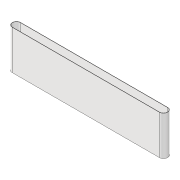
# Autodesk Inventor part: Band
Saved by Autodesk Inventor 2020 (Build 240168000, 168)
## iProperties
Created: 2020-03-18
Part Number: Band
Material: Generisch
Document SubType Name: Modeling
Designer: franz
Density: 1 g/cm^3
Appearance: Vorgabe
Author: franz
Autodesk Inventor part; units mm, degrees
ref_plane "YZ Plane" through (0, 0, 0) normal (1, 0, 0) x (0, 1, 0)
ref_plane "XZ Plane" through (0, 0, 0) normal (0, 1, 0) x (-1, 0, 0)
ref_plane "XY Plane" through (0, 0, 0) normal (0, 0, 1) x (1, 0, 0)
sketch "Skizze1" plane through (0, 0, 0) normal (0, 1, 0) x (-1, 0, 0)
  arc A0 (0, -40) -> (0, 40) centre (0, 0) ccw
  arc A1 (0, -43) -> (0, 43) centre (0, 0) ccw
  arc A2 (-1500, 40) -> (-1500, -40) centre (-1500, 0) ccw
  arc A3 (-1500, 43) -> (-1500, -43) centre (-1500, 0) ccw
  line L0 (0, 43) -> (-1500, 43)
  line L1 (-1500, 40) -> (0, 40)
  line L2 (0, -40) -> (-1500, -40)
  line L3 (-1500, -43) -> (0, -43)
  dimension "d0" = 80
  dimension "d1" = 86
  dimension "d2" = 80
  dimension "d3" = 86
  dimension "d4" = 1500
  constraints: 12 point on circle, 8 end point, 4 centre point, 4 coincident, 4 point on line, 4 tangent, 3 parallel, 1 horizontal
  measures "d0" diameter of A0
  measures "d1" diameter of A1
  measures "d2" diameter of A2
  measures "d3" diameter of A3
  measures "d4" distance of point (-1500, 0) point (0, 0)
extrude "Extrusion1" add sketch "Skizze1" along normal blind 340
